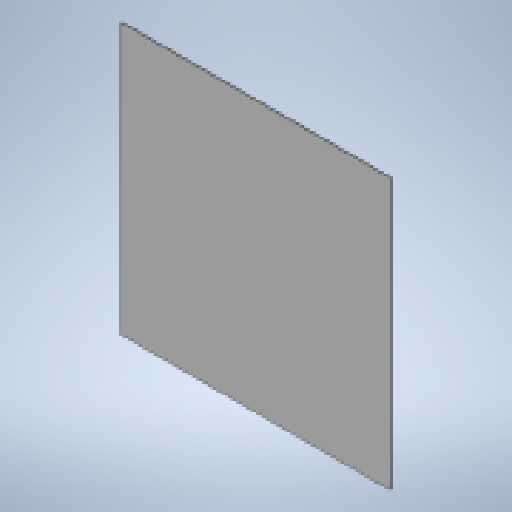
# Autodesk Inventor part: CH 1019 GBK shield
Saved by Autodesk Inventor 2026 (Build 300175000, 175)
## iProperties
Created: 2026-04-17
Part Number: CH 1019 GBK shield
Material: Steel
Document SubType Name: Sheet Metal
Designer: pokla
Density: 7.85 g/cm^3
Sheet Metal Rule: По умолчанию_мм
Appearance: Default
Mass: 69243.3 g
Surface Area: 44341.6 cm^2
Volume: 8820.8 cm^3
Flat Pattern Width: 148 cm
Flat Pattern Length: 149 cm
Flat Pattern Area: 22052 cm^2
Sheet Metal Width: 1480,000 мм
Sheet Metal Length: 1490,000 мм
Sheet Metal Area: 2205200,000 мм^2
Stock Number: 1318
Author: admin
Autodesk Inventor part; units mm, degrees
ref_plane "YZ Plane" through (0, 0, 0) normal (1, 0, 0) x (0, 1, 0)
ref_plane "XZ Plane" through (0, 0, 0) normal (0, 1, 0) x (-1, 0, 0)
ref_plane "XY Plane" through (0, 0, 0) normal (0, 0, 1) x (1, 0, 0)
sketch "Sketch1" plane through (0, 0, 0) normal (0, 0, 1) x (1, 0, 0)
  line L0 (740, -745) -> (-740, -745)
  line L1 (-740, -745) -> (-740, 745)
  line L2 (-740, 745) -> (740, 745)
  line L3 (740, 745) -> (740, -745)
  line L4 (740, -745) -> (-740, 745) construction
  line L5 (-740, -745) -> (740, 745) construction
  point P0 (0, 0)
  dimension "d0" = 1480
  dimension "d1" = 1490
  measures "d0" distance of L1.end L2.end
  measures "d1" distance of L0.end L1.end
extrude "Plate1" add sketch "Sketch1" along normal blind 4
sketch "Sketch2" plane through (0, 0, 0) normal (0, 0, -1) x (-1, 0, 0)
  line L0 (525.2603, -544.1907) -> (525.2603, -1005.879) construction
  line L1 (525.2603, -1005.879) -> (495.2603, -1005.879) construction
  line L2 (495.2603, -1005.879) -> (495.2603, -544.1907) construction
  line L3 (495.2603, -544.1907) -> (525.2603, -544.1907) construction
  line L4 (210.5058, -493) -> (210.5058, -590) projected
  line L5 (210.5058, -590) -> (206.5068, -590) projected
  line L6 (-289.6228, -493) -> (-289.6228, -590) projected
  line L7 (-289.6228, -590) -> (-293.6218, -590) projected
  ellipse E0 centre (-289.6228, 745) end of major axis (-289.6228, 775) minor radius 0.6803 (-289.6228, 715) -> (-289.6228, 775) ccw projected
  line L8 (-289.6228, 715) -> (-293.6218, 715) projected
  ellipse E1 centre (210.5058, 745) end of major axis (210.5058, 775) minor radius 0.6803 (210.5058, 715) -> (210.5058, 775) ccw projected
  line L9 (210.5058, 715) -> (206.5068, 715) projected
  line L10 (-739.3197, -489.5) -> (-710, -489.5) projected
  line L11 (-710, -489.5) -> (-710, -485.5) projected
  line L12 (-739.3197, 7.1667) -> (-710, 7.1667) projected
  line L13 (-710, 7.1667) -> (-710, 11.1667) projected
  line L14 (-739.3197, 503.8333) -> (-710, 503.8333) projected
  line L15 (-710, 503.8333) -> (-710, 507.8333) projected
  line L16 (710, -489.5) -> (710, -485.5) construction
  line L17 (710, 7.1667) -> (710, 11.1667) projected
  line L18 (710, 503.8333) -> (710, 507.8333) projected
  line L19 (710, -489.5) -> (710, -485.5) projected
  line L20 (710, 503.8333) -> (680, 503.8333)
  line L21 (710, 7.1667) -> (680, 7.1667)
  line L22 (710, -489.5) -> (680, -489.5)
  point P0 (0, 0)
  dimension "d6" = 30
  dimension "d7" = 30
  dimension "d8" = 30
  constraints: 6 end point, 3 horizontal, 4 other
  measures "d6" distance of L18.start L20.end
  measures "d7" distance of L17.start L21.end
  measures "d8" distance of L16.start L22.end
mark "Mark1"
equation "\"d0\" = Лист_ширина"
equation "\"d2\" = Thickness"
equation "\"BendRadius\" = Thickness"
equation "\"BendReliefWidth\" = Thickness"
equation "\"BendReliefDepth\" = 0.5 * Thickness"
equation "\"CornerReliefSize\" = 4 * Thickness"
equation "\"MinimumRemnant\" = 2 * Thickness"
equation "\"TransitionRadius\" = BendRadius"
equation "\"JacobiRadiusSize\" = BendRadius"
equation "\"GapSize\" = Thickness"
equation "\"Лист_ширина\" = 1480"
equation "\"Thickness\" = 4"
body "Solid1"
